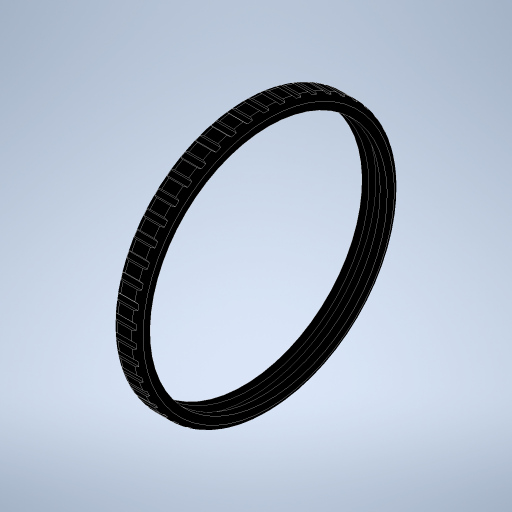
# Autodesk Inventor part: Neumatico
Saved by Autodesk Inventor 2023 (Build 270158000, 158)
## iProperties
Created: 2024-08-07
Part Number: Neumatico
Material: Generic
Document SubType Name: Modeling
Designer: LEGION
Density: 1 g/cm^3
Appearance: Default
Author: LEGION
Autodesk Inventor part; units mm, degrees
ref_plane "YZ Plane" through (0, 0, 0) normal (1, 0, 0) x (0, 1, 0)
ref_plane "XZ Plane" through (0, 0, 0) normal (0, 1, 0) x (-1, 0, 0)
ref_plane "XY Plane" through (0, 0, 0) normal (0, 0, 1) x (1, 0, 0)
sketch "Sketch1" plane through (0, 0, 0) normal (0, 0, 1) x (1, 0, 0)
  line L0 (-1.6, 37.35) -> (1.6, 37.35)
  line L1 (1.6, 37.35) -> (1.6, 35.75)
  line L2 (1.6, 35.75) -> (-1.6, 35.75)
  line L3 (-1.6, 35.75) -> (-1.6, 37.35)
  line L4 (1.6, 37.35) -> (2, 37.35)
  line L5 (3.6, 35.75) -> (3.6, 33.75)
  line L6 (3.6, 33.75) -> (1.6, 33.75)
  line L7 (1.6, 33.75) -> (1.6, 37.35)
  line L8 (-1.6, 37.35) -> (-2, 37.35)
  line L9 (-3.6, 35.75) -> (-3.6, 33.75)
  line L10 (-3.6, 33.75) -> (-1.6, 33.75)
  line L11 (-1.6, 33.75) -> (-1.6, 37.35)
  arc A0 (3.6, 35.75) -> (2, 37.35) centre (2, 35.75) ccw
  arc A1 (-2, 37.35) -> (-3.6, 35.75) centre (-2, 35.75) ccw
  line L12 (0, 0) -> (3.0314, 0)
  point P0 (3.6, 37.35)
  point P1 (-3.6, 37.35)
  point P2 (-1.6, 35.75)
  point P3 (1.6, 35.75)
  dimension "d0" = 35.75
  dimension "d1" = 1.6
  dimension "d2" = 3.2
  dimension "d3" = 1.6
  dimension "d4" = 2
  dimension "d5" = 2
  dimension "d6" = 3.6
  dimension "d7" = 3.6
  dimension "d8" = 1.6
  dimension "d10" = 2
  constraints: 26 end point, 6 parallel, 4 horizontal, 4 point on circle, 4 point on line, 4 tangent, 3 perpendicular, 2 centre point, 1 equal radius
  measures "d0" distance from line of L12.start L2
  measures "d1" distance of L2.end L0.start
  measures "d2" distance of L0.start L0.end
  measures "d3" distance from line of L12.start L1
  measures "d4" distance of L5.end L6.end
  measures "d5" distance of L9.end L10.end
  measures "d6" distance of point (-3.6, 37.35) L9.end
  measures "d7" distance of point (3.6, 37.35) L5.end
  measures "d8" radius of A0
  measures "d10" distance between parallel lines of L2 L6
revolve "Revolution1" add sketch "Sketch1" angle 360 about axis through (0, 0, 0) along (1, 0, 0)
sketch "Sketch2" plane through (3.6, 0, 0) normal (1, 0, 0) x (0, 0, -1)
  line L0 (-1, 37.35) -> (1, 37.35)
  line L1 (1, 37.35) -> (1, 37.35)
  line L2 (0.7, 37.05) -> (-0.7, 37.05)
  line L3 (-1, 37.35) -> (-1, 37.35)
  circle A0 centre (0, 0) radius 37.35 projected
  line L4 (1, 37.35) -> (0.7, 37.05)
  line L5 (-1, 37.35) -> (-0.7, 37.05)
  point P0 (1, 37.05)
  point P1 (-1, 37.05)
  point P2 (0.987, 37.337)
  point P3 (-0.987, 37.337)
  dimension "d12" = 1
  dimension "d13" = 2
  dimension "d14" = 0.3
  dimension "d15" = 0.3
  dimension "d16" = 0.3
  dimension "d17" = 0.3
  dimension "d18" = 0.3
  constraints: 12 end point, 4 point on line, 2 parallel, 1 horizontal, 1 perpendicular, 1 tangent
  measures "d12" distance from line of point (0, 0) L1
  measures "d13" distance between parallel lines of L1 L3
  measures "d14" distance of L0.end point (1, 37.05)
  measures "d15" distance of L1.end point (1, 37.05)
  measures "d16" distance of L2.start point (1, 37.05)
  measures "d17" distance of L3.start point (-1, 37.05)
  measures "d18" distance of L2.end point (-1, 37.05)
extrude "Extrusion1" cut sketch "Sketch2" against normal blind 10 contours A0 L4 L2 L5 picked at (0, 37.15)
pattern_circular "Circular Pattern1" count 50 over 360 about axis through (-10, 0, 0) along (1, 0, 0) of "Extrusion1"
equation "\"d3\" = 0.5 * d2"
equation "\"d12\" = 0.5 * d13"
equation "\"d16\" = d15"
equation "\"d18\" = d17"
body "Solid1"
